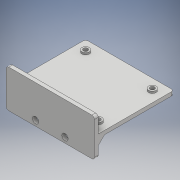
# Autodesk Inventor part: Eletronica - suporte210N06
Saved by Autodesk Inventor 2017 (Build 210142000, 142)
## iProperties
Created: 2020-10-10
Part Number: Eletronica - suporte210N06
Material: Generic
Document SubType Name: Modeling
Designer: ale
Density: 1 g/cm^3
Appearance: Default
Author: ale
Autodesk Inventor part; units mm, degrees
ref_plane "YZ Plane" through (0, 0, 0) normal (1, 0, 0) x (0, 1, 0)
ref_plane "XZ Plane" through (0, 0, 0) normal (0, 1, 0) x (-1, 0, 0)
ref_plane "XY Plane" through (0, 0, 0) normal (0, 0, 1) x (1, 0, 0)
sketch "Sketch1" plane through (0, 0, 0) normal (0, 0, 1) x (1, 0, 0)
  line L0 (-35, 30) -> (35, 30)
  line L1 (35, 30) -> (35, -30)
  line L2 (35, -30) -> (-35, -30)
  line L3 (-35, -30) -> (-35, 30)
  line L4 (-35, 30) -> (35, -30) construction
  line L5 (35, 30) -> (-35, -30) construction
  point P0 (0, 0)
  dimension "d0" = 70
  dimension "d1" = 60
  constraints: 12 end point, 2 midpoint, 2 parallel, 1 horizontal, 1 perpendicular
  measures "d0" distance of L1.end L2.end
  measures "d1" distance of L0.end L1.end
extrude "Extrusion1" add sketch "Sketch1" along normal blind 3
sketch "Sketch2" plane through (0, 0, 3) normal (0, 0, 1) x (1, 0, 0)
  line L0 (-30, 25) -> (30, 25)
  line L1 (30, 25) -> (30, -25)
  line L2 (30, -25) -> (-30, -25)
  line L3 (-30, -25) -> (-30, 25)
  line L4 (-30, 25) -> (30, -25) construction
  line L5 (30, 25) -> (-30, -25) construction
  line L6 (-26.5, 21.5) -> (26.5, 21.5)
  line L7 (26.5, 21.5) -> (26.5, -21.5)
  line L8 (26.5, -21.5) -> (-26.5, -21.5)
  line L9 (-26.5, -21.5) -> (-26.5, 21.5)
  line L10 (-26.5, 21.5) -> (26.5, -21.5) construction
  line L11 (26.5, 21.5) -> (-26.5, -21.5) construction
  circle A0 centre (-26.5, 21.5) radius 3
  circle A1 centre (26.5, 21.5) radius 3
  circle A2 centre (26.5, -21.5) radius 3
  circle A3 centre (-26.5, -21.5) radius 3
  point P0 (0, 0)
  dimension "d4" = 60
  dimension "d5" = 50
  dimension "d6" = 53
  dimension "d7" = 43
  dimension "d8" = 6
  dimension "d9" = 6
  dimension "d10" = 6
  dimension "d11" = 6
  constraints: 24 end point, 4 centre point, 4 coincident, 4 midpoint, 4 parallel, 2 horizontal, 2 perpendicular
  measures "d4" distance of L1.end L2.end
  measures "d5" distance of L0.end L1.end
  measures "d6" distance of L7.end L8.end
  measures "d7" distance of L6.end L7.end
  measures "d8" diameter of A0
  measures "d9" diameter of A1
  measures "d10" diameter of A2
  measures "d11" diameter of A3
extrude "Extrusion2" add sketch "Sketch2" along normal blind 1.5 contours L9 A0 L6 | L6 A0 L9 | A1 L7 L6 | L6 L7 A1 | A3 L8 L9 | L9 L8 A3 | A2 L8 L7 | L7 L8 A2
sketch "Sketch3" plane through (-26.5, 21.5, 4.5) normal (0, 0, 1) x (1, 0, 0)
  circle A0 centre (53, 0) radius 3 projected
  circle A1 centre (53, -43) radius 3 projected
  circle A2 centre (0, -43) radius 3 projected
  point P0 (26.5, -21.5)
  point P1 (0, 0)
  constraints: 3 coincident
hole "Hole1" at (-26.5, 21.5, 4.5) at (26.5, 21.5, 4.5) at (26.5, -21.5, 4.5) at (-26.5, -21.5, 4.5) direction (0, 0, -1) diameter 3.5 end through all
sketch "Sketch4" plane through (-35, -30, 0) normal (0, -1, 0) x (1, 0, 0)
  line L0 (0, 0) -> (0, 3) projected
  line L1 (0, 1.5) -> (70, 1.5)
  line L2 (70, 0) -> (0, 0) projected
  line L3 (0, 16.5) -> (70, 16.5)
  line L4 (70, 16.5) -> (70, -13.5)
  line L5 (70, -13.5) -> (0, -13.5)
  line L6 (0, -13.5) -> (0, 16.5)
  line L7 (0, 16.5) -> (70, -13.5) construction
  line L8 (70, 16.5) -> (0, -13.5) construction
  point P0 (35, 0)
  point P1 (35, 1.5)
  dimension "d21" = 70
  dimension "d22" = 30
  constraints: 14 end point, 4 midpoint, 3 parallel, 1 horizontal, 1 perpendicular
  measures "d21" distance of L4.end L5.end
  measures "d22" distance of L3.end L4.end
extrude "Extrusion3" add sketch "Sketch4" along normal blind 3
chamfer "Chamfer1" distance 5 angle 45 1 edges at (0, -30, 0)
sketch "Sketch5" plane through (-35, -30, 0) normal (0, 1, 0) x (1, 0, 0)
  line L0 (0, 13.5) -> (70, 13.5) projected
  line L1 (0, 13.5) -> (0, 5) projected
  point P0 (35, 0)
  point P1 (23.3333, 9.25)
  point P2 (46.6667, 9.25)
  dimension "d28" = 4.25
  dimension "d29" = 4.25
  dimension "d30" = 23.3333
  dimension "d31" = 46.6667
  measures "d28" distance from line of L0 point (46.667, 9.25)
  measures "d29" distance from line of point (23.333, 9.25) L0
  measures "d30" distance from line of point (23.333, 9.25) L1
  measures "d31" distance from line of point (46.667, 9.25) L1
hole "Hole2" at (-11.6667, -30, -9.25) at (11.6667, -30, -9.25) direction (0, -1, 0) diameter 5 end through all
fillet "Fillet1" radius 2 6 edges at (35, -31.5, -13.5) (35, 30, 1.5) (35, -31.5, 16.5) (-35, -31.5, 16.5) (-35, 30, 1.5) (-35, -31.5, -13.5)
body "Solid1"
